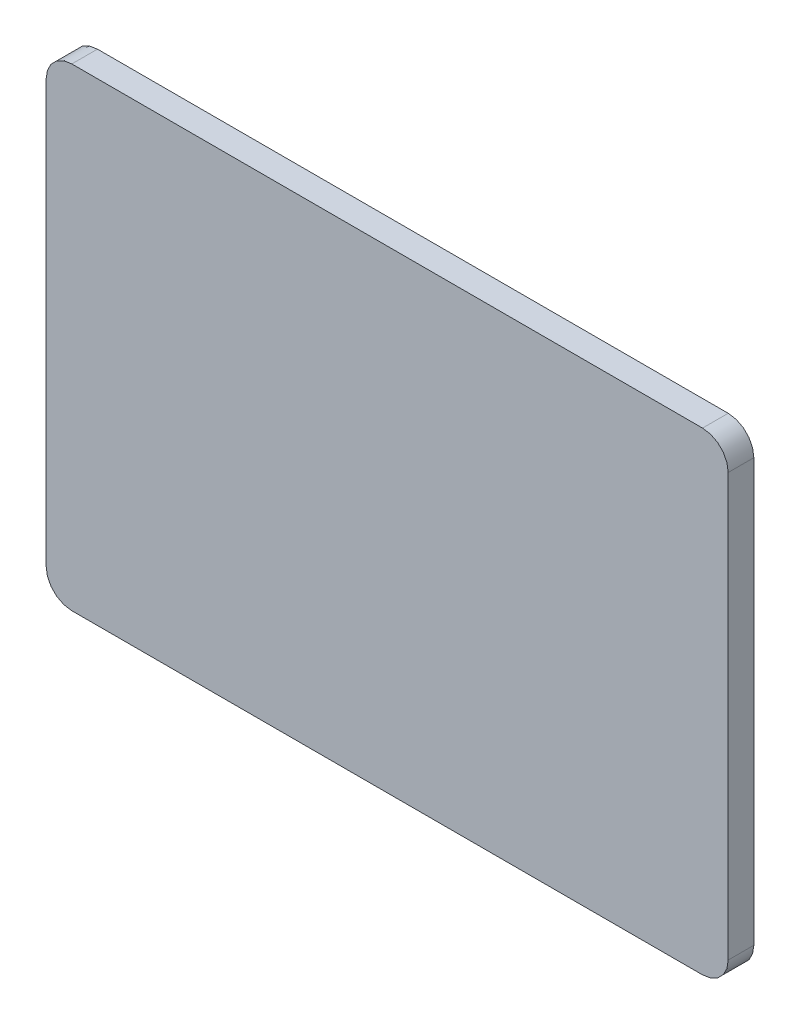
# Autodesk Inventor part: Frame_Lid
Saved by Autodesk Inventor 2023 (Build 270158000, 158)
## iProperties
Created: 2023-10-08
Part Number: Frame_Lid
Material: Generic
Document SubType Name: Modeling
Designer: a laptop
Density: 1 g/cm^3
Appearance: Default
Author: a laptop
Autodesk Inventor part; units mm, degrees
ref_plane "YZ Plane" through (0, 0, 0) normal (1, 0, 0) x (0, 1, 0)
ref_plane "XZ Plane" through (0, 0, 0) normal (0, 1, 0) x (-1, 0, 0)
ref_plane "XY Plane" through (0, 0, 0) normal (0, 0, 1) x (1, 0, 0)
sketch "Sketch1" plane through (0, 0, 0) normal (0, 0, 1) x (1, 0, 0)
  line L0 (2, 0) -> (51.18, 0)
  line L1 (53.18, 2) -> (53.18, 34.924)
  line L2 (51.18, 36.924) -> (2, 36.924)
  line L3 (0, 34.924) -> (0, 2)
  arc A0 (2, 36.924) -> (0, 34.924) centre (2, 34.924) ccw
  arc A1 (0, 2) -> (2, 0) centre (2, 2) ccw
  arc A2 (51.18, 0) -> (53.18, 2) centre (51.18, 2) ccw
  arc A3 (53.18, 34.924) -> (51.18, 36.924) centre (51.18, 34.924) ccw
  point P0 (0, 0)
  point P1 (53.18, 36.924)
  point P2 (53.18, 0)
  point P3 (0, 36.924)
  dimension "d0" = 36.924
  dimension "d1" = 53.18
  dimension "d2" = 2
  constraints: 8 end point, 8 point on circle, 8 point on line, 8 tangent, 4 centre point, 3 equal radius, 2 parallel, 1 horizontal, 1 perpendicular
  measures "d0" distance of point (53.18, 0) point (53.18, 36.924)
  measures "d1" distance of point (53.18, 36.924) point (0, 36.924)
  measures "d2" radius of A0
extrude "Extrusion1" add sketch "Sketch1" along normal blind 2
sketch "Sketch2" plane through (0, 0, 2) normal (0, 0, 1) x (1, 0, 0)
  point P0 (0, 0)
body "Solid1"
